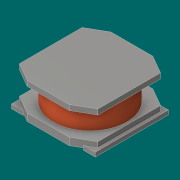
# Autodesk Inventor part: SRN4018
Saved by Autodesk Inventor 2016 (Build 200138000, 138)
## iProperties
Created: 2016-03-02
Part Number: SRN4018
Material: ABS Plastic
Document SubType Name: Modeling
Designer: Sawaiz
Density: 1.06 g/cm^3
Appearance: Smooth - Medium Gray
Author: Sawaiz
Autodesk Inventor part; units mm, degrees
ref_plane "YZ Plane" through (0, 0, 0) normal (1, 0, 0) x (0, 1, 0)
ref_plane "XZ Plane" through (0, 0, 0) normal (0, 1, 0) x (-1, 0, 0)
ref_plane "XY Plane" through (0, 0, 0) normal (0, 0, 1) x (1, 0, 0)
sketch "Sketch1" plane through (0, 0, 0) normal (0, 0, 1) x (1, 0, 0)
  line L0 (1.75, -2) -> (-1.75, -2)
  line L1 (-1.75, -2) -> (-1.75, 2)
  line L2 (-1.75, 2) -> (1.75, 2)
  line L3 (1.75, 2) -> (1.75, -2)
  line L4 (1.75, -2) -> (-1.75, 2) construction
  line L5 (-1.75, -2) -> (1.75, 2) construction
  line L6 (-2, -1) -> (-2, 1)
  line L7 (-2, 1) -> (-1.4948, 1.875)
  line L8 (-1.4948, 1.875) -> (1.4948, 1.875)
  line L9 (1.4948, 1.875) -> (2, 1)
  line L10 (2, 1) -> (2, -1)
  line L11 (2, -1) -> (1.4948, -1.875)
  line L12 (1.4948, -1.875) -> (-1.4948, -1.875)
  line L13 (-1.4948, -1.875) -> (-2, -1)
  line L14 (-2, -1) -> (2, 1) construction
  line L15 (-2, 1) -> (2, -1) construction
  point P0 (0, 0)
  point P1 (0, 0)
  dimension "d0" = 3.5
  dimension "d1" = 4
  dimension "d2" = 4
  dimension "d3" = 3.75
  dimension "d6" = 150
  dimension "d7" = 150
  dimension "d8" = 2
  constraints: 32 end point, 5 midpoint, 5 parallel, 3 equal length, 3 perpendicular, 1 horizontal, 1 vertical
  measures "d0" distance of L1.end L2.end
  measures "d1" distance of L0.end L1.end
  measures "d2" distance between parallel lines of L6 L10
  measures "d3" distance between parallel lines of L12 L8
  measures "d6" angle of L6 L13
  measures "d7" angle of L6 L7
  measures "d8" distance of L9.end L10.end
extrude "Extrusion1" add sketch "Sketch1" along normal blind 1.6 contours L11 L12 L13 L1 L7 L8 L9 L3 | L3 L9 L10 L11 | L13 L6 L7 L1
sketch "Sketch2" plane through (0, 0, 0) normal (0, 0, -1) x (-1, 0, 0)
  line L0 (2, -1) -> (2, 1) projected
  line L1 (2, 1) -> (1.4948, 1.875) projected
  line L2 (1.4948, 1.875) -> (-1.4948, 1.875) projected
  line L3 (-1.4948, 1.875) -> (-2, 1) projected
  line L4 (-2, 1) -> (-2, -1) projected
  line L5 (-2, -1) -> (-1.4948, -1.875) projected
  line L6 (-1.4948, -1.875) -> (1.4948, -1.875) projected
  line L7 (1.4948, -1.875) -> (2, -1) projected
  line L8 (-1.75, -2) -> (1.75, -2)
  line L9 (1.75, -2) -> (1.75, 2)
  line L10 (1.75, 2) -> (-1.75, 2)
  line L11 (-1.75, 2) -> (-1.75, -2)
  line L12 (-1.75, -2) -> (1.75, 2) construction
  line L13 (1.75, -2) -> (-1.75, 2) construction
  point P0 (0, 0)
  dimension "d11" = 3.5
  dimension "d12" = 4
  constraints: 12 end point, 2 midpoint, 2 parallel, 1 horizontal, 1 perpendicular
  measures "d11" distance of L10.end L9.end
  measures "d12" distance of L9.end L8.end
extrude "Extrusion2" add sketch "Sketch2" along normal blind 0.2 contours L9 L8 L11 L5 L6 L7 | L7 L6 L5 L11 L3 L2 L1 L9 | L1 L2 L3 L11 L10 L9
sketch "Sketch3" plane through (0, 0, 0) normal (0, 0, -1) x (-1, 0, 0)
  line L0 (-1.75, -1.433) -> (-1.75, 1.433) projected
  line L1 (-1.75, 1.433) -> (-2, 1) projected
  line L2 (-2, 1) -> (-2, -1) projected
  line L3 (-2, -1) -> (-1.75, -1.433) projected
  line L4 (1.75, 1.433) -> (1.75, -1.433) projected
  line L5 (1.75, -1.433) -> (2, -1) projected
  line L6 (2, -1) -> (2, 1) projected
  line L7 (2, 1) -> (1.75, 1.433) projected
  point P0 (0, 0)
extrude "Extrusion3" add sketch "Sketch3" along normal up to surface (0.2 mm away)
sketch "Sketch4" plane through (0, 0, 0) normal (0, 1, 0) x (-1, 0, 0)
  line L0 (-2, 1.6) -> (-2, -0.2) projected
  line L1 (-1.4948, 1.6) -> (-2, 1.6) projected
  line L2 (-1.4948, 0) -> (-1.4948, 1.6) projected
  line L3 (-1.75, 0) -> (-1.4948, 0) projected
  line L4 (-1.75, -0.2) -> (-1.75, 0) projected
  line L5 (-1.75, -0.2) -> (-2, -0.2) projected
  line L6 (1.4948, 0) -> (1.75, 0) projected
  line L7 (1.4948, 0) -> (1.4948, 1.6) projected
  line L8 (2, 1.6) -> (1.4948, 1.6) projected
  line L9 (2, -0.2) -> (2, 1.6) projected
  line L10 (2, -0.2) -> (1.75, -0.2) projected
  line L11 (1.75, 0) -> (1.75, -0.2) projected
  line L12 (-3.75, 1.35) -> (-1.75, 1.35)
  line L13 (-1.75, 1.35) -> (-1.75, 0.25)
  line L14 (-1.75, 0.25) -> (-3.75, 0.25)
  line L15 (-3.75, 0.25) -> (-3.75, 1.35)
  line L16 (-1.75, -0.2) -> (1.75, -0.2) projected
  line L17 (0, -0.56) -> (0, 1.96) projected
  point P0 (0, 0)
  dimension "d18" = 0.25
  dimension "d19" = 0.25
  dimension "d21" = 2
  dimension "d22" = 0.25
  constraints: 8 end point, 2 parallel, 1 horizontal, 1 perpendicular
  measures "d18" distance between parallel lines of L1 L12
  measures "d19" distance between parallel lines of L14 L3
  measures "d21" distance of L12.start L12.end
  measures "d22" distance between parallel lines of L0 L13
revolve "Revolution1" cut sketch "Sketch4" angle 360 about axis through (0, 0, -10) along (0, 0, 1) contours L12 L13 L14 L0 | L0 L14 L15 L12
sketch "Sketch5" plane through (0, 0, -0.2) normal (0, 0, -1) x (-1, 0, 0)
  line L0 (-1.75, -2) -> (1.75, -2) projected
  line L1 (1.75, -2) -> (1.75, -1.433) projected
  line L2 (2, -1) -> (1.75, -1.433) projected
  line L3 (2, 1) -> (2, -1) projected
  line L4 (1.75, 1.433) -> (2, 1) projected
  line L5 (1.75, 1.433) -> (1.75, 2) projected
  line L6 (1.75, 2) -> (-1.75, 2) projected
  line L7 (-1.75, 2) -> (-1.75, 1.433) projected
  line L8 (-2, 1) -> (-1.75, 1.433) projected
  line L9 (-2, -1) -> (-2, 1) projected
  line L10 (-1.75, -1.433) -> (-2, -1) projected
  line L11 (-1.75, -1.433) -> (-1.75, -2) projected
  line L12 (2, -1.433) -> (-2, -1.433)
  line L13 (-2, -1.433) -> (-2, 1.433)
  line L14 (-2, 1.433) -> (2, 1.433)
  line L15 (2, 1.433) -> (2, -1.433)
  line L16 (2, -1.433) -> (-2, 1.433) construction
  line L17 (-2, -1.433) -> (2, 1.433) construction
  point P0 (0, 0)
  constraints: 12 end point, 2 midpoint, 2 parallel, 1 collinear, 1 horizontal, 1 perpendicular, 1 point on line
extrude "Extrusion4" cut sketch "Sketch5" against normal blind 0.1 contours L12 L13 L10 | L10 L9 L8 L14 L4 L3 L2 L12 | L2 L15 L12 | L13 L14 L8 | L4 L14 L15
body "Solid1"
